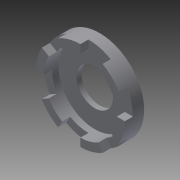
# Autodesk Inventor part: Stator
Saved by Autodesk Inventor 2018.2 (Build 222227000, 227)
## iProperties
Created: 2018-02-02
Part Number: Stator
Material: Generic
Document SubType Name: Modeling
Designer: Rus
Density: 1 g/cm^3
Appearance: Default
Author: Rus
Autodesk Inventor part; units mm, degrees
ref_plane "YZ Plane" through (0, 0, 0) normal (1, 0, 0) x (0, 1, 0)
ref_plane "XZ Plane" through (0, 0, 0) normal (0, 1, 0) x (-1, 0, 0)
ref_plane "XY Plane" through (0, 0, 0) normal (0, 0, 1) x (1, 0, 0)
sketch "Sketch1" plane through (0, 0, 0) normal (0, 0, 1) x (1, 0, 0)
  circle A0 centre (0, 0) radius 38.1
  circle A1 centre (0, 0) radius 19.05
  dimension "d0" = 76.2
  dimension "d1" = 38.1
  constraints: 2 centre point, 2 coincident
  measures "d0" diameter of A0
  measures "d1" diameter of A1
extrude "Extrusion1" add sketch "Sketch1" along normal blind 5.08
sketch "Sketch2" plane through (0, 0, 0) normal (0, 0, -1) x (-1, 0, 0)
  circle A0 centre (0, 0) radius 46.5667
  circle A1 centre (0, 0) radius 38.1 projected
  dimension "d8" = 8.4667
  constraints: 1 centre point, 1 coincident
  measures "d8" radial gap between concentric circles of A0 A1
extrude "Extrusion2" add sketch "Sketch2" against normal blind 20.2142
sketch "Sketch3" plane through (0, 0, 20.2142) normal (0, 0, 1) x (1, 0, 0)
  circle A0 centre (0, 0) radius 46.5667 construction
  arc A1 (23.2833, 40.3279) -> (0, 46.5667) centre (0, 0) ccw
  line L0 (0, 0) -> (23.2833, 40.3279) construction
  line L1 (0, 0) -> (0, 46.5667) construction
  circle A2 centre (0, 0) radius 38.1 projected
  circle A3 centre (0, 0) radius 46.5667 projected
  circle A4 centre (0, 0) radius 38.1 projected
  line L2 (0, 38.1) -> (0, 46.5667)
  line L3 (19.05, 32.9956) -> (23.2833, 40.3279)
  arc A5 (19.05, 32.9956) -> (0, 38.1) centre (0, 0) ccw
  dimension "d9" = 30
  constraints: 8 end point, 5 point on circle, 2 centre point, 2 coincident, 2 point on line, 1 collinear, 1 vertical, 1 vertical alignment, 3 other
  measures "d9" angle of L0 L1
extrude "Extrusion3" cut sketch "Sketch3" against normal blind 8.4667 contours L3 A2 L2 A1
pattern_circular "Circular Pattern1" count 6 over 360 about axis through (0, 0, 0) along (0, 0, 1) of "Extrusion3"
body "Solid1"
